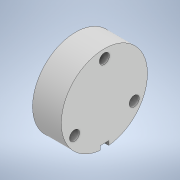
# Autodesk Inventor part: 711124
Saved by Autodesk Inventor 2022 (Build 260153000, 153)
## iProperties
Created: 2021-10-21
Part Number: 711124
Material: Типовые
Document SubType Name: Modeling
Designer: RaNSiD
Density: 1 g/cm^3
Appearance: По умолчанию
Author: RaNSiD
Autodesk Inventor part; units mm, degrees
ref_plane "YZ Plane" through (0, 0, 0) normal (1, 0, 0) x (0, 1, 0)
ref_plane "XZ Plane" through (0, 0, 0) normal (0, 1, 0) x (-1, 0, 0)
ref_plane "XY Plane" through (0, 0, 0) normal (0, 0, 1) x (1, 0, 0)
sketch "Эскиз1" plane through (0, 0, 0) normal (0, 0, 1) x (1, 0, 0)
  line L0 (0, 0) -> (20, 0)
  line L1 (20, 0) -> (20, 30)
  line L2 (20, 30) -> (0, 30)
  line L3 (0, 30) -> (0, 0)
  dimension "d0" = 20
  dimension "d1" = 30
  constraints: 8 end point, 2 parallel, 1 horizontal, 1 perpendicular
  measures "d0" distance of L2.end L1.end
  measures "d1" distance of L1.end L0.end
revolve "Вращение1" add sketch "Эскиз1" angle 360 about axis through (0, 0, 0) along (1, 0, 0)
sketch "Эскиз2" plane through (0, 0, 0) normal (-1, 0, 0) x (0, 0, 1)
  point P0 (0, 0)
  point P1 (0, 24)
  point P2 (-20.7846, -12)
  point P3 (20.7846, -12)
  dimension "d3" = 24
  dimension "d6" = 360
  constraints: 4 other
  measures "d3" distance of point (0, 0) point (0, 24)
hole "Отверстие1" at (0, 24, 0) at (0, -12, -20.7846) at (0, -12, 20.7846) direction (1, 0, 0) diameter 7 end through all counterbore diameter 9 counterbore depth 5
sketch "Эскиз3" plane through (0, 0, 0) normal (-1, 0, 0) x (0, 0, 1)
  point P0 (0, 0)
  point P1 (0, 0)
  constraints: 1 coincident
hole "Отверстие2" at (0, 0, 0) direction (1, 0, 0) diameter 30 depth 16 countersink diameter 34 countersink angle 90
sketch "Эскиз4" plane through (0, 0, 0) normal (-1, 0, 0) x (0, 0, 1)
  circle A0 centre (0, 0) radius 30 construction
  line L0 (-3, -27) -> (3, -27)
  line L1 (3, -27) -> (3, -29.8496)
  line L2 (-3, -29.8496) -> (-3, -27)
  arc A1 (-3, -29.8496) -> (3, -29.8496) centre (0, 0) ccw
  point P0 (0, -27)
  dimension "d22" = 6
  dimension "d23" = 27
  constraints: 6 end point, 4 point on circle, 1 centre point, 1 concentric, 1 horizontal, 1 midpoint, 1 parallel, 1 perpendicular, 1 vertical alignment
  measures "d22" distance of L0.start L0.end
  measures "d23" distance of point (0, -27) point (0, 0)
extrude "Выдавливание1" cut sketch "Эскиз4" against normal blind 20
